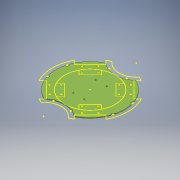
# Autodesk Inventor part: motherboard
Saved by Autodesk Inventor 2020 (Build 240168000, 168)
## iProperties
Created: 2024-11-03
Part Number: motherboard
Material: Медь
Document SubType Name: Modeling
Designer: Ivan
Density: 8.94 g/cm^3
Appearance: Оливково-зеленый
Author: Ivan
Autodesk Inventor part; units mm, degrees
ref_plane "YZ Plane" through (0, 0, 0) normal (1, 0, 0) x (0, 1, 0)
ref_plane "XZ Plane" through (0, 0, 0) normal (0, 1, 0) x (-1, 0, 0)
ref_plane "XY Plane" through (0, 0, 0) normal (0, 0, 1) x (1, 0, 0)
sketch "Эскиз1" plane through (0, 2, -127) normal (0, 1, 0) x (1, 0, 0)
  circle A0 centre (-90.3481, -100.1076) radius 1.5
  circle A1 centre (90.3481, -153.8924) radius 1.5
  circle A2 centre (-90.3481, -153.8924) radius 1.5
  circle A3 centre (90.3481, -100.1076) radius 1.5
  circle A4 centre (51.0265, -155.3991) radius 1.5
  circle A5 centre (-67.0849, -171.4575) radius 1.5
  circle A6 centre (-44.4575, -59.9151) radius 1.5
  circle A7 centre (51.0265, -98.6009) radius 1.5
  circle A8 centre (28.3991, -75.9735) radius 1.5
  circle A9 centre (-67.0849, -82.5425) radius 1.5
  circle A10 centre (-28.3991, -178.0265) radius 1.5
  circle A11 centre (28.3991, -178.0265) radius 1.5
  circle A12 centre (67.0849, -171.4575) radius 1.5
  circle A13 centre (-51.0265, -155.3991) radius 1.5
  circle A14 centre (-28.3991, -75.9735) radius 1.5
  circle A15 centre (67.0849, -82.5425) radius 1.5
  circle A16 centre (44.4575, -59.9151) radius 1.5
  circle A17 centre (-51.0265, -98.6009) radius 1.5
  circle A18 centre (-44.4575, -194.0849) radius 1.5
  circle A19 centre (44.4575, -194.0849) radius 1.5
  arc A20 (-36.9892, -29.8002) -> (36.9892, -29.8002) centre (0, 0) ccw
  arc A21 (-36.9892, -29.8002) -> (-48.2758, -34.8835) centre (0, -127) ccw
  line L0 (-48.2758, -34.8835) -> (-38.4471, -44.7123)
  line L1 (-38.4471, -44.7123) -> (-82.2877, -88.5529)
  line L2 (-82.2877, -88.5529) -> (-92.1165, -78.7242)
  arc A22 (-92.1165, -78.7242) -> (-92.1165, -175.2758) centre (0, -127) ccw
  line L3 (-92.1165, -175.2758) -> (-82.2877, -165.4471)
  line L4 (-82.2877, -165.4471) -> (-38.4471, -209.2877)
  line L5 (-38.4471, -209.2877) -> (-48.2758, -219.1165)
  arc A23 (-48.2758, -219.1165) -> (-36.9892, -224.1998) centre (0, -127) ccw
  arc A24 (36.9892, -224.1998) -> (-36.9892, -224.1998) centre (0, -254) ccw
  arc A25 (36.9892, -224.1998) -> (48.2758, -219.1165) centre (0, -127) ccw
  line L6 (48.2758, -219.1165) -> (38.4471, -209.2877)
  line L7 (38.4471, -209.2877) -> (82.2877, -165.4471)
  line L8 (82.2877, -165.4471) -> (92.1165, -175.2758)
  arc A26 (92.1165, -175.2758) -> (92.1165, -78.7242) centre (0, -127) ccw
  line L9 (92.1165, -78.7242) -> (82.2877, -88.5529)
  line L10 (82.2877, -88.5529) -> (38.4471, -44.7123)
  line L11 (38.4471, -44.7123) -> (48.2758, -34.8835)
  arc A27 (48.2758, -34.8835) -> (36.9892, -29.8002) centre (0, -127) ccw
  line L12 (-67.0849, -82.5425) -> (-51.0265, -98.6009) construction
  circle A28 centre (0, -127) radius 69.3873
  line L13 (-62.0891, -96.0236) -> (-51.0265, -107.0862)
  line L14 (-51.0265, -107.0862) -> (-19.9138, -75.9735)
  line L15 (-19.9138, -75.9735) -> (-30.9764, -64.9109)
  line L16 (-51.0265, -146.9138) -> (-62.0891, -157.9764)
  line L17 (-19.9138, -178.0265) -> (-51.0265, -146.9138)
  line L18 (-30.9764, -189.0891) -> (-19.9138, -178.0265)
  line L19 (19.9138, -178.0265) -> (30.9764, -189.0891)
  line L20 (51.0265, -146.9138) -> (19.9138, -178.0265)
  line L21 (62.0891, -157.9764) -> (51.0265, -146.9138)
  line L22 (51.0265, -107.0862) -> (62.0891, -96.0236)
  line L23 (19.9138, -75.9735) -> (51.0265, -107.0862)
  line L24 (30.9764, -64.9109) -> (19.9138, -75.9735)
  point P0 (-59.0557, -90.5717)
sketch "Эскиз2" plane through (0, 2, 127) normal (0, 1, 0) x (1, 0, 0)
  circle A0 centre (0, 127) radius 104
  line L0 (-92.1165, 78.7242) -> (-82.2877, 88.5529)
  line L1 (-82.2877, 88.5529) -> (-38.4471, 44.7123)
  line L2 (-38.4471, 44.7123) -> (-48.2758, 34.8835)
  line L3 (48.2758, 34.8835) -> (38.4471, 44.7123)
  line L4 (38.4471, 44.7123) -> (82.2877, 88.5529)
  line L5 (82.2877, 88.5529) -> (92.1165, 78.7242)
  line L6 (82.2877, 165.4471) -> (38.4471, 209.2877)
  line L7 (38.4471, 209.2877) -> (48.2758, 219.1165)
  line L8 (92.1165, 175.2758) -> (82.2877, 165.4471)
  line L9 (-48.2758, 219.1165) -> (-38.4471, 209.2877)
  line L10 (-38.4471, 209.2877) -> (-82.2877, 165.4471)
  line L11 (-82.2877, 165.4471) -> (-92.1165, 175.2758)
sketch "Эскиз3_1" plane through (0, 2, 127) normal (0, 1, 0) x (1, 0, 0)
  circle A0 centre (-23.8556, 50.0189) radius 1.5
  circle A1 centre (23.8556, 50.0189) radius 1.5
  circle A2 centre (-23.8556, 203.9811) radius 1.5
  circle A3 centre (23.8556, 203.9811) radius 1.5
  point P0 (0, 127)
sketch "Эскиз3" plane through (0, 0, 0) normal (0, 1, 0) x (-1, 0, 0)
  arc A0 (-36.9892, 97.1998) -> (36.9892, 97.1998) centre (0, 127) ccw projected
  line L0 (38.4471, 82.2877) -> (48.2758, 92.1165) projected
  line L1 (-48.2758, 92.1165) -> (-38.4471, 82.2877) projected
  arc A1 (-38.4471, 82.2877) -> (38.4471, 82.2877) centre (0, 133.1293) ccw
  circle A2 centre (0, 0) radius 69.3873 construction
  circle A3 centre (90.3481, 26.8924) radius 1.5 projected
  line L2 (82.2877, 38.4471) -> (38.4471, 82.2877) projected
  arc A4 (92.1165, -48.2758) -> (92.1165, 48.2758) centre (0, 0) ccw projected
  line L3 (104, 0) -> (-104.6293, 0) construction
  arc A5 (48.6356, -91.927) -> (-48.6356, -91.927) centre (0, -133.1293) ccw
  circle A6 centre (0, 0) radius 104
  arc A7 (38.4471, 82.2877) -> (48.5783, 91.8595) centre (0, 133.1293) ccw
  arc A8 (-48.6356, 91.927) -> (-38.4471, 82.2877) centre (0, 133.1293) ccw
  circle A9 centre (0, 0) radius 94.2655
  circle A10 centre (90.3481, -26.8924) radius 1.5 projected
  circle A11 centre (-90.3481, -26.8924) radius 1.5 projected
  circle A12 centre (-90.3481, 26.8924) radius 1.5 projected
  circle A13 centre (90.3481, 26.8924) radius 4
  circle A14 centre (90.3481, -26.8924) radius 4
  circle A15 centre (-90.3481, -26.8924) radius 4
  circle A16 centre (-90.3481, 26.8924) radius 4
  circle A17 centre (67.0849, 44.4575) radius 1.5 projected
  circle A18 centre (44.4575, 67.0849) radius 1.5 projected
  circle A19 centre (28.3991, 51.0265) radius 1.5 projected
  circle A20 centre (51.0265, 28.3991) radius 1.5 projected
  circle A21 centre (51.0265, -28.3991) radius 1.5 projected
  circle A22 centre (67.0849, -44.4575) radius 1.5 projected
  circle A23 centre (44.4575, -67.0849) radius 1.5 projected
  circle A24 centre (23.8556, 76.9811) radius 1.5 projected
  circle A25 centre (-23.8556, 76.9811) radius 1.5 projected
  circle A26 centre (23.8556, 76.9811) radius 4
  circle A27 centre (-23.8556, 76.9811) radius 4
  circle A28 centre (23.8556, -76.9811) radius 4
  circle A29 centre (-23.8556, -76.9811) radius 4
  point P0 (0, 69.3873)
  point P1 (60.3674, 60.3674)
  point P2 (38.4471, -82.2877)
  point P3 (-38.4471, -82.2877)
  point P4 (-41.4193, 84.6784)
  point P5 (-89.1259, 30.7011)
  point P6 (-91.4077, 23.0352)
  point P7 (-91.4077, -23.0352)
  point P8 (-89.1259, -30.7011)
  point P9 (-41.4193, -84.6784)
  point P10 (41.4193, -84.6784)
  point P11 (89.1259, -30.7011)
  point P12 (91.4077, -23.0352)
  point P13 (91.4077, 23.0352)
  point P14 (89.1259, 30.7011)
  point P15 (41.4193, 84.6784)
  point P16 (-27.6425, -75.6929)
  point P17 (-22.1541, -73.3611)
  point P18 (22.1541, -73.3611)
  point P19 (27.6425, -75.6929)
  point P20 (27.6425, 75.6929)
  point P21 (22.1541, 73.3611)
  point P22 (-22.1541, 73.3611)
  point P23 (-27.6425, 75.6929)
  dimension "d1" = 8
  constraints: 16 point on circle, 13 centre point, 10 coincident, 5 equal radius, 5 symmetric about line, 2 end point, 1 horizontal, 1 midpoint, 1 point on line, 1 vertical alignment, 7 other
  measures "d1" diameter of A13
extrude "Выдавливание1" add sketch "Эскиз3" along normal blind 2 contours A1 A27 A26 A7 A9 A13 A14 A5 A28 A29 A15 A16 A8
hole "Отверстие1" at (-44.4575, 2, -67.0849) at (-67.0849, 2, -44.4575) at (-28.3991, 2, -51.0265) at (-51.0265, 2, -28.3991) at (44.4575, 2, -67.0849) at (67.0849, 2, -44.4575) at (28.3991, 2, -51.0265) at (51.0265, 2, -28.3991) at (51.0265, 2, 28.3991) at (67.0849, 2, 44.4575) at (44.4575, 2, 67.0849) at (28.3991, 2, 51.0265) at (-51.0265, 2, 28.3991) at (-28.3991, 2, 51.0265) at (-44.4575, 2, 67.0849) at (-67.0849, 2, 44.4575) direction (0, -1, 0) diameter 3 end through all
fillet "Сопряжение1" radius 4 16 edges at (-89.1259, 1, -30.7011) (-91.4077, 1, -23.0352) (-89.1259, 1, 30.7011) (-91.4077, 1, 23.0352) (91.4077, 1, -23.0352) (91.4077, 1, 23.0352) (89.1259, 1, 30.7011) (89.1259, 1, -30.7011) (-27.6425, 1, 75.6929) (-22.1541, 1, 73.3611) (22.1541, 1, 73.3611) (27.6425, 1, 75.6929) (-27.6425, 1, -75.6929) (-22.1541, 1, -73.3611) (27.6425, 1, -75.6929) (22.1541, 1, -73.3611)
sketch "Эскиз5" plane through (0, 2, 0) normal (0, 1, 0) x (1, 0, 0)
  line L0 (-15.1, 31) -> (15.1, 31) construction
  line L1 (15.1, 31) -> (15.1, -31) construction
  line L2 (15.1, -31) -> (-15.1, -31) construction
  line L3 (-15.1, -31) -> (-15.1, 31) construction
  line L4 (-15.1, 31) -> (15.1, -31) construction
  circle A0 centre (0, 0) radius 69.3873 projected
  arc A1 (92.1165, -48.2758) -> (92.1165, 48.2758) centre (0, 0) ccw projected
  arc A2 (-92.1117, 20.0355) -> (-92.1117, -20.0355) centre (0, 0) ccw projected
  dimension "d12" = 62
  dimension "d13" = 30.2
  constraints: 10 end point, 6 coincident, 2 parallel, 1 horizontal, 1 midpoint, 1 perpendicular
  measures "d12" distance of L0.end L1.end
  measures "d13" distance of L0.start L0.end
hole "Отверстие2" at (-15.1, 2, -31) at (15.1, 2, -31) at (15.1, 2, 31) at (-15.1, 2, 31) direction (0, -1, 0) diameter 3 end through all
